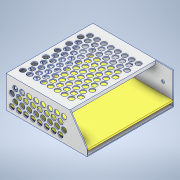
# Autodesk Inventor part: Power Supply
Saved by Autodesk Inventor 2021 (Build 250183000, 183)
## iProperties
Created: 2021-04-06
Part Number: Power Supply
Material: Generic
Document SubType Name: Modeling
Designer: Andrew
Density: 1 g/cm^3
Appearance: Default
power_supply_side_mount_len: 27.500 mm
Author: Andrew
Autodesk Inventor part; units mm, degrees
ref_plane "YZ Plane" through (0, 0, 0) normal (1, 0, 0) x (0, 1, 0)
ref_plane "XZ Plane" through (0, 0, 0) normal (0, 1, 0) x (-1, 0, 0)
ref_plane "XY Plane" through (0, 0, 0) normal (0, 0, 1) x (1, 0, 0)
sketch "Sketch1" plane through (0, 0, 0) normal (0, 0, 1) x (1, 0, 0)
  line L0 (0, 0) -> (70, 0)
  line L1 (55, 27.5) -> (0, 27.5)
  line L2 (0, 27.5) -> (0, 0)
  line L3 (55, 27.5) -> (70, 5.5)
  line L4 (70, 5.5) -> (70, 0)
  line L5 (55, 27.5) -> (55, 24.5)
  line L6 (55, 24.5) -> (54.25, 24.5)
  line L7 (54.25, 24.5) -> (54.25, 26.75)
  line L8 (54.25, 26.75) -> (0.75, 26.75)
  line L9 (0.75, 26.75) -> (0.75, 0.75)
  line L10 (0.75, 0.75) -> (70, 0.75)
  line L11 (70, 5.5) -> (1.25, 5.5)
  line L12 (1.25, 5.5) -> (1.25, 3.93)
  line L13 (1.25, 3.93) -> (70, 3.93)
  line L14 (70, 3.93) -> (70, 5.5)
  line L15 (55, 27.5) -> (70, 27.5)
  line L16 (70, 27.5) -> (70, 5.5)
  dimension "d0" = 27.5
  dimension "d1" = 70
  dimension "d2" = 55
  dimension "d3" = 5.5
  dimension "d8" = 3
  dimension "d9" = 0.75
  dimension "d10" = 0.75
  dimension "d11" = 0.75
  dimension "d12" = 0.75
  dimension "d13" = 0.5
  dimension "d14" = 1.57
  constraints: 34 end point, 6 perpendicular, 5 parallel, 3 horizontal, 2 vertical, 1 point on line
  measures "d0" distance of L1.end L0.start
  measures "d1" distance of L0.start L0.end
  measures "d2" distance of L1.start L1.end
  measures "d3" distance of L3.end L0.end
  measures "d8" distance of L1.start L5.end
  measures "d9" distance between parallel lines of L8 L1
  measures "d10" distance between parallel lines of L9 L2
  measures "d11" distance between parallel lines of L0 L10
  measures "d12" distance between parallel lines of L5 L7
  measures "d13" distance between parallel lines of L9 L12
  measures "d14" distance between parallel lines of L11 L13
extrude "Extrusion1" add sketch "Sketch1" along normal mid plane 75 contours L2 L1 L5 L6 L7 L8 L9 L10 L4 L0 | L10 L9 L8 L7 L6 L5 L3 L11 L12 L13 L4 | L13 L12 L11 L4
extrude "Extrusion4" add sketch "Sketch1" against normal up to surface (37.5 mm away) contours L15 L16 L3
extrude "Extrusion2" cut sketch "Sketch1" along normal mid plane 73.5 contours L10 L9 L8 L7 L6 L5 L3 L11 L12 L13 L4 | L15 L16 L3 | L13 L12 L11 L4
extrude "Extrusion3" add sketch "Sketch1" along normal mid plane 73 separate body contours L13 L12 L11 L4
sketch "Sketch2" plane through (0, 27.5, -37.5) normal (0, 1, 0) x (1, 0, 0)
  circle A0 centre (5, -65.5) radius 2.25
  circle A1 centre (8, -60.5) radius 2.25
  circle A2 centre (11, -65.5) radius 2.25 construction
  line L0 (8, -60.5) -> (8, -65.5) construction
  line L1 (0, 0) -> (0, -75) projected
  line L2 (55, -75) -> (0, -75) projected
  point P0 (0, -37.5)
  dimension "d19" = 4.5
  dimension "d20" = 4.5
  dimension "d21" = 4.5
  dimension "d23" = 6
  dimension "d24" = 5
  dimension "d25" = 5
  dimension "d26" = 9.5
  constraints: 3 centre point, 2 end point, 2 horizontal alignment, 1 symmetric about line, 1 vertical
  measures "d19" diameter of A0
  measures "d20" diameter of A1
  measures "d21" diameter of A2
  measures "d23" distance of A2.centre A0.centre
  measures "d24" vertical distance of L0.start A0.centre
  measures "d25" distance from line of A0.centre L1
  measures "d26" distance from line of A0.centre L2
extrude "Extrusion5" add sketch "Sketch2" against normal up to surface (0.75 mm away) separate body contours A0
pattern_linear "Rectangular Pattern1" count 8 spacing 6 along (1, 0, 0) bodies 3
extrude "Extrusion6" add sketch "Sketch2" against normal up to surface (0.75 mm away) separate body contours A1
pattern_linear "Rectangular Pattern2" count 8 spacing 6 along (1, 0, 0) bodies 4
pattern_linear "Rectangular Pattern3" count 6 spacing 10 along (0, 0, -1) bodies 4 3
combine bodies "Combine1" operation type subtract main body 1 bodies to subtract 3 4
sketch "Sketch3" plane through (0, 0, 37.5) normal (0, 0, 1) x (1, 0, 0)
  circle A0 centre (5, 5) radius 2.25
  circle A1 centre (8, 10) radius 2.25
  circle A2 centre (11, 5) radius 2.25 construction
  line L0 (8, 10) -> (8, 5) construction
  line L1 (0, 0) -> (70, 0) projected
  line L2 (0, 27.5) -> (0, 0) projected
  dimension "d40" = 4.5
  dimension "d41" = 4.5
  dimension "d42" = 4.5
  dimension "d43" = 6
  dimension "d44" = 5
  dimension "d45" = 5
  dimension "d46" = 5
  constraints: 3 centre point, 2 end point, 2 horizontal alignment, 1 symmetric about line, 1 vertical
  measures "d40" diameter of A0
  measures "d41" diameter of A1
  measures "d42" diameter of A2
  measures "d43" distance of A2.centre A0.centre
  measures "d44" vertical distance of L0.start A0.centre
  measures "d45" distance from line of L1 A0.centre
  measures "d46" distance from line of L2 A0.centre
extrude "Extrusion7" add sketch "Sketch3" against normal up to surface (0.75 mm away) separate body contours A0
extrude "Extrusion8" add sketch "Sketch3" against normal up to surface (0.75 mm away) contours A1 bodies 5
pattern_linear "Rectangular Pattern4" count 8 spacing 6 along (1, 0, 0) count 2 spacing 10 along (0, 1, 0) bodies 5
combine bodies "Combine2" operation type subtract main body 1 bodies to subtract 5
sketch "Sketch4" plane through (0, 0, 37.5) normal (-1, 0, 0) x (0, 0, 1)
  circle A0 centre (-19, 7.5) radius 2.25 construction
  circle A1 centre (-14, 10.5) radius 2.25
  circle A2 centre (-9, 7.5) radius 2.25
  line L0 (-14, 10.5) -> (-14, 7.5) construction
  line L1 (0, 27.5) -> (0, 0) projected
  line L2 (0, 0) -> (-75, 0) projected
  point P0 (-37.5, 0)
  dimension "d57" = 4.5
  dimension "d58" = 4.5
  dimension "d59" = 4.5
  dimension "d60" = 10
  dimension "d61" = 3
  dimension "d62" = 9
  dimension "d63" = 7.5
  constraints: 3 centre point, 2 end point, 2 horizontal alignment, 1 symmetric about line, 1 vertical
  measures "d57" diameter of A0
  measures "d58" diameter of A1
  measures "d59" diameter of A2
  measures "d60" distance of A2.centre A0.centre
  measures "d61" vertical distance of L0.start A0.centre
  measures "d62" distance from line of L1 A2.centre
  measures "d63" distance from line of L2 A2.centre
extrude "Extrusion9" add sketch "Sketch4" against normal up to surface (0.75 mm away) separate body contours A2
extrude "Extrusion10" add sketch "Sketch4" against normal up to surface (0.75 mm away) separate body contours A1
pattern_linear "Rectangular Pattern5" count 3 spacing 6 along (0, 1, 0) bodies 6
pattern_linear "Rectangular Pattern6" count 6 spacing 10 along (0, 0, -1) bodies 6
pattern_linear "Rectangular Pattern7" count 2 spacing 6 along (0, 1, 0) bodies 7
pattern_linear "Rectangular Pattern8" count 5 spacing 10 along (0, 0, -1) bodies 7
combine bodies "Combine3" operation type subtract main body 1 bodies to subtract 6 7
sketch "Power Supply Side Mount" plane through (0, 0, -37.5) normal (0, 0, -1) x (-1, 0, 0)
  circle A0 centre (-61.5, 15) radius 1.25
  circle A1 centre (-34, 15) radius 1.25
  line L0 (0, 27.5) -> (-70, 27.5) projected
  line L1 (0, 0) -> (0, 27.5) projected
  dimension "d80" = 2.5
  dimension "d81" = 2.5
  dimension "d82" = 12.5
  dimension "d83" = 34
  dimension "power_supply_side_mount_len" = 27.5
  constraints: 2 centre point, 1 horizontal alignment
  measures "d80" diameter of A0
  measures "d81" diameter of A1
  measures "d82" distance from line of A0.centre L0
  measures "d83" distance from line of L1 A1.centre
  measures "power_supply_side_mount_len" distance of A1.centre A0.centre
extrude "Extrusion11" cut sketch "Power Supply Side Mount" against normal up to surface (0.75 mm away) bodies 1
thread "Thread1" size "M2.5x0.45" class "6H" standard "ANSI Metric M Profile" full length
thread "Thread2" size "M2.5x0.45" class "6H" standard "ANSI Metric M Profile" full length
sketch "Sketch6" plane through (0, 0, 37.5) normal (0, -1, 0) x (1, 0, 0)
  circle A0 centre (4, -37) radius 1.25
  circle A1 centre (54, -37) radius 1.25
  line L0 (0, 0) -> (70, 0) projected
  line L1 (0, 0) -> (0, -75) projected
  point P0 (0, -37.5)
  dimension "d91" = 37
  dimension "d92" = 2.5
  dimension "d93" = 2.5
  dimension "d94" = 4
  dimension "d95" = 50
  constraints: 2 centre point, 1 horizontal alignment
  measures "d91" distance from line of L0 A0.centre
  measures "d92" diameter of A0
  measures "d93" diameter of A1
  measures "d94" distance from line of A0.centre L1
  measures "d95" distance of A1.centre A0.centre
extrude "Extrusion12" cut sketch "Sketch6" against normal up to surface (0.75 mm away) bodies 1
thread "Thread3" size "M2.5x0.45" class "6H" standard "ANSI Metric M Profile" full length
thread "Thread4" size "M2.5x0.45" class "6H" standard "ANSI Metric M Profile" full length
body "Solid1"
body "Solid2"
